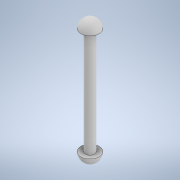
# Autodesk Inventor part: Pino da dobradiça
Saved by Autodesk Inventor 2021 (Build 250183000, 183)
## iProperties
Created: 2021-08-09
Part Number: Pino da dobradiça
Material: Generic
Document SubType Name: Modeling
Designer: guilh
Density: 1 g/cm^3
Appearance: Default
Author: guilh
Autodesk Inventor part; units mm, degrees
ref_plane "YZ Plane" through (0, 0, 0) normal (1, 0, 0) x (0, 1, 0)
ref_plane "XZ Plane" through (0, 0, 0) normal (0, 1, 0) x (-1, 0, 0)
ref_plane "XY Plane" through (0, 0, 0) normal (0, 0, 1) x (1, 0, 0)
sketch "Sketch1" plane through (0, 0, 0) normal (0, 1, 0) x (-1, 0, 0)
  circle A0 centre (0, 0) radius 3
  dimension "d0" = 6
  constraints: 1 centre point, 1 coincident
  measures "d0" diameter of A0
extrude "Extrusion1" add sketch "Sketch1" along normal blind 70
sketch "Sketch2" plane through (0, 70, 0) normal (0, 1, 0) x (1, 0, 0)
  point P0 (0, 0)
sketch "Sketch3" plane through (0, 0, 0) normal (1, 0, 0) x (0, 1, 0)
  line L0 (0, 0) -> (0, -9)
  line L1 (0, -3) -> (0, 3) projected
  line L2 (0, 0) -> (-9, 0)
  arc A0 (-9, 0) -> (0, -9) centre (0, 0) ccw
  line L3 (70, -3) -> (70, 3) projected
  arc A1 (70, -9) -> (79, 0) centre (70, 0) ccw
  line L4 (79, 0) -> (70, 0)
  line L5 (70, -9) -> (70, 0)
  dimension "d3" = 9
  dimension "d4" = 9
  dimension "d5" = 9
  constraints: 8 end point, 4 point on circle, 2 centre point, 2 horizontal, 1 coincident, 1 collinear, 1 midpoint, 1 perpendicular, 1 point on line
  measures "d3" distance of L0.start L0.end
  measures "d4" distance of L0.start L2.end
  measures "d5" radius of A1
revolve "Revolution1" add sketch "Sketch3" angle 360 about axis through (0, 79, 0) along (0, -1, 0)
sketch "Sketch4" plane through (0, 0, 0) normal (1, 0, 0) x (0, 1, 0)
  line L0 (0, -10.1336) -> (-13.8396, -10.1336)
  line L1 (-13.8396, -10.1336) -> (-13.8396, 13.3764)
  line L2 (-13.8396, 13.3764) -> (0, 13.3764)
  line L3 (0, 13.3764) -> (0, -10.1336)
  line L4 (70, 9) -> (70, -9) projected
  line L5 (70, -9) -> (70, 12.4499)
  line L6 (70, 12.4499) -> (83.9063, 12.4499)
  line L7 (83.9063, 12.4499) -> (83.9063, -12.3341)
  line L8 (83.9063, -12.3341) -> (70, -9)
  point P0 (0, 0)
  constraints: 16 end point, 5 perpendicular, 1 horizontal, 1 vertical
extrude "Extrusion2" cut sketch "Sketch4" along normal mid plane 20
sketch "Sketch5" plane through (0, 0, 0) normal (1, 0, 0) x (0, 1, 0)
  line L0 (0, 0) -> (0, -6)
  line L1 (0, -3) -> (0, 3) projected
  line L2 (0, 0) -> (-6, 0)
  arc A0 (-6, 0) -> (0, -6) centre (0, 0) ccw
  line L3 (70, -3) -> (70, 3) projected
  line L4 (70, 0) -> (76, 0)
  line L5 (70, 0) -> (70, -6)
  arc A1 (70, -6) -> (76, 0) centre (70, 0) ccw
  dimension "d9" = 6
  dimension "d10" = 6
  dimension "d11" = 6
  dimension "d12" = 6
  constraints: 8 end point, 4 point on circle, 2 centre point, 2 coincident, 2 horizontal, 1 collinear, 1 midpoint, 1 point on line, 1 vertical
  measures "d9" distance of L0.start L0.end
  measures "d10" distance of L0.start L2.end
  measures "d11" distance of L4.start L4.end
  measures "d12" distance of L4.start L5.end
revolve "Revolution2" add sketch "Sketch5" angle 360 about axis through (0, 70, 0) along (0, 1, 0)
body "Solid1"
